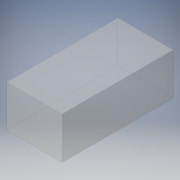
# Autodesk Inventor part: catapultMaxVolume
Saved by Autodesk Inventor 2016 SP1 (Build 200210100, 210)
## iProperties
Created: 2016-01-12
Part Number: catapultMaxVolume
Material: Polycarbonate, Clear
Document SubType Name: Modeling
Designer: steele
Density: 1.2 g/cm^3
Appearance: Polycarbonate - Clear
Author: steele
Autodesk Inventor part; units mm, degrees
ref_plane "YZ Plane" through (0, 0, 0) normal (1, 0, 0) x (0, 1, 0)
ref_plane "XZ Plane" through (0, 0, 0) normal (0, 1, 0) x (-1, 0, 0)
ref_plane "XY Plane" through (0, 0, 0) normal (0, 0, 1) x (1, 0, 0)
sketch "Sketch2" plane through (0, 0, 0) normal (0, 1, 0) x (-1, 0, 0)
  line L0 (254, 508) -> (-254, 508)
  line L1 (-254, 508) -> (-254, -508)
  line L2 (-254, -508) -> (254, -508)
  line L3 (254, -508) -> (254, 508)
  line L4 (254, 508) -> (-254, -508) construction
  line L5 (-254, 508) -> (254, -508) construction
  point P0 (0, 0)
  dimension "d4" = 508
  dimension "d5" = 1016
  constraints: 12 end point, 2 midpoint, 2 parallel, 1 horizontal, 1 perpendicular
  measures "d4" distance of L0.start L0.end
  measures "d5" distance of L2.end L0.start
extrude "Extrusion1" add sketch "Sketch2" along normal blind 381
equation "\"d4\" = width"
equation "\"d5\" = length"
equation "\"d6\" = height"
equation "\"width\" = -length + 0.5 * perimeter"
equation "\"length\" = 1016"
equation "\"height\" = 381"
equation "\"perimeter\" = 3048"
body "Solid1"
